Autodesk Inventor part; units mm, degrees
(part 4 of 4)
sketch "Эскиз12" plane through (0, 0, 5) normal (0, 0, 1) x (1, 0, 0)
  arc A0 (45.1929, -106.1976) -> (44.4998, -103.5049) centre (42.2719, -105.5139) ccw projected
  arc A1 (-3.3547, -38.1199) -> (-21.9349, -33.766) centre (-14.404, -43.4501) ccw projected
  line L0 (-21.9349, -33.766) -> (-22.5081, -34.2402) projected
  line L1 (-22.5081, -34.2402) -> (-23.0514, -34.7484) projected
  line L2 (-23.0514, -34.7484) -> (-23.3602, -34.9338) projected
  line L3 (-23.3602, -34.9338) -> (-23.5194, -34.9702) projected
  line L4 (-23.5194, -34.9702) -> (-23.6529, -34.9806) projected
  line L5 (-23.6529, -34.9806) -> (-23.7727, -34.9768) projected
  line L6 (-23.7727, -34.9768) -> (-23.8833, -34.9636) projected
  line L7 (-23.8833, -34.9636) -> (-24.0859, -34.9174) projected
  line L8 (-24.0859, -34.9174) -> (-24.2711, -34.8524) projected
  line L9 (-24.2711, -34.8524) -> (-24.4437, -34.7734) projected
  line L10 (-24.4437, -34.7734) -> (-24.6063, -34.683) projected
  line L11 (-24.6063, -34.683) -> (-24.9077, -34.4748) projected
  line L12 (-24.9077, -34.4748) -> (-25.1895, -34.2439) projected
  line L13 (-25.1895, -34.2439) -> (-25.5122, -34.0611) projected
  line L14 (-25.5122, -34.0611) -> (-25.8619, -33.9111) projected
  line L15 (-25.8619, -33.9111) -> (-26.2315, -33.7867) projected
  line L16 (-26.2315, -33.7867) -> (-26.6177, -33.685) projected
  line L17 (-26.6177, -33.685) -> (-27.0185, -33.6047) projected
  line L18 (-27.0185, -33.6047) -> (-27.4325, -33.5452) projected
  line L19 (-27.4325, -33.5452) -> (-27.8584, -33.5059) projected
  line L20 (-27.8584, -33.5059) -> (-28.295, -33.4867) projected
  line L21 (-28.295, -33.4867) -> (-28.7415, -33.4875) projected
  line L22 (-28.7415, -33.4875) -> (-29.0823, -33.5012) projected
  line L23 (-29.0823, -33.5012) -> (-30.1782, -35.3504) projected
  line L24 (-30.1782, -35.3504) -> (-30.0266, -35.6559) projected
  line L25 (-30.0266, -35.6559) -> (-29.813, -36.0479) projected
  line L26 (-29.813, -36.0479) -> (-29.5865, -36.4218) projected
  line L27 (-29.5865, -36.4218) -> (-29.3476, -36.7765) projected
  line L28 (-29.3476, -36.7765) -> (-29.0966, -37.111) projected
  line L29 (-29.0966, -37.111) -> (-28.8338, -37.4241) projected
  line L30 (-28.8338, -37.4241) -> (-28.5592, -37.7141) projected
  line L31 (-28.5592, -37.7141) -> (-28.2726, -37.9785) projected
  line L32 (-28.2726, -37.9785) -> (-27.9731, -38.2133) projected
  line L33 (-27.9731, -38.2133) -> (-27.6579, -38.4086) projected
  line L34 (-27.6579, -38.4086) -> (-27.32, -38.545) projected
  line L35 (-27.32, -38.545) -> (-26.9927, -38.7094) projected
  line L36 (-26.9927, -38.7094) -> (-26.8353, -38.8087) projected
  line L37 (-26.8353, -38.8087) -> (-26.6832, -38.9221) projected
  line L38 (-26.6832, -38.9221) -> (-26.5372, -39.0534) projected
  line L39 (-26.5372, -39.0534) -> (-26.3994, -39.209) projected
  line L40 (-26.3994, -39.209) -> (-26.3347, -39.2997) projected
  line L41 (-26.3347, -39.2997) -> (-26.2739, -39.4029) projected
  line L42 (-26.2739, -39.4029) -> (-26.2189, -39.5249) projected
  line L43 (-26.2189, -39.5249) -> (-26.1744, -39.6821) projected
  line L44 (-26.1744, -39.6821) -> (-26.1888, -40.0421) projected
  line L45 (-26.1888, -40.0421) -> (-26.3737, -40.7626) projected
  line L46 (-26.3737, -40.7626) -> (-26.5146, -41.493) projected
  line L47 (-26.5146, -41.493) -> (-26.6554, -41.8246) projected
  line L48 (-26.6554, -41.8246) -> (-26.7629, -41.9477) projected
  line L49 (-26.7629, -41.9477) -> (-26.8648, -42.0345) projected
  line L50 (-26.8648, -42.0345) -> (-26.9639, -42.1018) projected
  line L51 (-26.9639, -42.1018) -> (-27.0611, -42.1561) projected
  line L52 (-27.0611, -42.1561) -> (-27.2522, -42.2379) projected
  line L53 (-27.2522, -42.2379) -> (-27.4403, -42.2942) projected
  line L54 (-27.4403, -42.2942) -> (-27.6263, -42.3317) projected
  line L55 (-27.6263, -42.3317) -> (-27.811, -42.3542) projected
  line L56 (-27.811, -42.3542) -> (-28.1772, -42.3629) projected
  line L57 (-28.1772, -42.3629) -> (-28.5409, -42.3417) projected
  line L58 (-28.5409, -42.3417) -> (-28.9094, -42.3835) projected
  line L59 (-28.9094, -42.3835) -> (-29.2805, -42.4677) projected
  line L60 (-29.2805, -42.4677) -> (-29.6526, -42.5842) projected
  line L61 (-29.6526, -42.5842) -> (-30.0249, -42.729) projected
  line L62 (-30.0249, -42.729) -> (-30.3963, -42.8997) projected
  line L63 (-30.3963, -42.8997) -> (-30.7662, -43.0948) projected
  line L64 (-30.7662, -43.0948) -> (-31.1338, -43.3134) projected
  line L65 (-31.1338, -43.3134) -> (-31.4984, -43.5545) projected
  line L66 (-31.4984, -43.5545) -> (-31.8591, -43.8176) projected
  line L67 (-31.8591, -43.8176) -> (-32.1268, -44.029) projected
  line L68 (-32.1268, -44.029) -> (-31.9265, -46.1692) projected
  line L69 (-31.9265, -46.1692) -> (-31.6243, -46.3272) projected
  line L70 (-31.6243, -46.3272) -> (-31.221, -46.5188) projected
  line L71 (-31.221, -46.5188) -> (-30.8181, -46.6881) projected
  line L72 (-30.8181, -46.6881) -> (-30.4163, -46.8347) projected
  line L73 (-30.4163, -46.8347) -> (-30.0166, -46.9578) projected
  line L74 (-30.0166, -46.9578) -> (-29.6199, -47.0566) projected
  line L75 (-29.6199, -47.0566) -> (-29.2273, -47.1298) projected
  line L76 (-29.2273, -47.1298) -> (-28.84, -47.1753) projected
  line L77 (-28.84, -47.1753) -> (-28.4598, -47.1892) projected
  line L78 (-28.4598, -47.1892) -> (-28.0899, -47.1619) projected
  line L79 (-28.0899, -47.1619) -> (-27.7364, -47.0736) projected
  line L80 (-27.7364, -47.0736) -> (-27.3749, -47.0142) projected
  line L81 (-27.3749, -47.0142) -> (-27.1893, -47.0021) projected
  line L82 (-27.1893, -47.0021) -> (-26.9995, -47.0044) projected
  line L83 (-26.9995, -47.0044) -> (-26.8043, -47.0248) projected
  line L84 (-26.8043, -47.0248) -> (-26.6014, -47.0697) projected
  line L85 (-26.6014, -47.0697) -> (-26.4957, -47.1051) projected
  line L86 (-26.4957, -47.1051) -> (-26.3859, -47.1528) projected
  line L87 (-26.3859, -47.1528) -> (-26.2696, -47.2192) projected
  line L88 (-26.2696, -47.2192) -> (-26.1412, -47.3202) projected
  line L89 (-26.1412, -47.3202) -> (-25.9413, -47.6199) projected
  line L90 (-25.9413, -47.6199) -> (-25.6674, -48.3115) projected
  line L91 (-25.6674, -48.3115) -> (-25.352, -48.9853) projected
  line L92 (-25.352, -48.9853) -> (-25.2711, -49.3363) projected
  line L93 (-25.2711, -49.3363) -> (-25.2857, -49.499) projected
  line L94 (-25.2857, -49.499) -> (-25.3171, -49.6291) projected
  line L95 (-25.3171, -49.6291) -> (-25.3576, -49.7418) projected
  line L96 (-25.3576, -49.7418) -> (-25.4044, -49.8429) projected
  line L97 (-25.4044, -49.8429) -> (-25.5109, -50.0214) projected
  line L98 (-25.5109, -50.0214) -> (-25.63, -50.1775) projected
  line L99 (-25.63, -50.1775) -> (-25.7585, -50.3172) projected
  line L100 (-25.7585, -50.3172) -> (-25.8946, -50.4439) projected
  line L101 (-25.8946, -50.4439) -> (-26.1858, -50.6662) projected
  line L102 (-26.1858, -50.6662) -> (-26.4925, -50.8629) projected
  line L103 (-26.4925, -50.8629) -> (-26.7661, -51.1133) projected
  line L104 (-26.7661, -51.1133) -> (-27.0168, -51.3996) projected
  line L105 (-27.0168, -51.3996) -> (-27.2493, -51.7125) projected
  line L106 (-27.2493, -51.7125) -> (-27.4654, -52.0484) projected
  line L107 (-27.4654, -52.0484) -> (-27.6656, -52.4049) projected
  line L108 (-27.6656, -52.4049) -> (-27.8501, -52.7802) projected
  line L109 (-27.8501, -52.7802) -> (-28.0191, -53.1731) projected
  line L110 (-28.0191, -53.1731) -> (-28.1723, -53.5824) projected
  line L111 (-28.1723, -53.5824) -> (-28.3095, -54.0073) projected
  line L112 (-28.3095, -54.0073) -> (-28.4018, -54.3356) projected
  line L113 (-28.4018, -54.3356) -> (-26.9818, -55.9493) projected
  line L114 (-26.9818, -55.9493) -> (-26.6444, -55.8996) projected
  line L115 (-26.6444, -55.8996) -> (-26.2055, -55.8175) projected
  line L116 (-26.2055, -55.8175) -> (-25.78, -55.7177) projected
  line L117 (-25.78, -55.7177) -> (-25.3688, -55.6001) projected
  line L118 (-25.3688, -55.6001) -> (-24.9731, -55.4648) projected
  line L119 (-24.9731, -55.4648) -> (-24.5941, -55.3116) projected
  line L120 (-24.5941, -55.3116) -> (-24.2334, -55.14) projected
  line L121 (-24.2334, -55.14) -> (-23.8934, -54.9491) projected
  line L122 (-23.8934, -54.9491) -> (-23.5776, -54.7369) projected
  line L123 (-23.5776, -54.7369) -> (-23.2944, -54.4974) projected
  line L124 (-23.2944, -54.4974) -> (-23.0603, -54.2182) projected
  line L125 (-23.0603, -54.2182) -> (-22.8028, -53.9577) projected
  line L126 (-22.8028, -53.9577) -> (-22.6598, -53.8387) projected
  line L127 (-22.6598, -53.8387) -> (-22.5048, -53.7291) projected
  line L128 (-22.5048, -53.7291) -> (-22.3349, -53.6308) projected
  line L129 (-22.3349, -53.6308) -> (-22.1443, -53.5479) projected
  line L130 (-22.1443, -53.5479) -> (-22.0381, -53.5144) projected
  line L131 (-22.0381, -53.5144) -> (-21.9211, -53.4885) projected
  line L132 (-21.9211, -53.4885) -> (-21.788, -53.4739) projected
  line L133 (-21.788, -53.4739) -> (-21.6248, -53.4801) projected
  line L134 (-21.6248, -53.4801) -> (-21.2869, -53.605) projected
  line L135 (-21.2869, -53.605) -> (-20.6588, -54.0036) projected
  line L136 (-20.6588, -54.0036) -> (-20.0076, -54.3632) projected
  line L137 (-20.0076, -54.3632) -> (-19.7358, -54.5996) projected
  line L138 (-19.7358, -54.5996) -> (-19.652, -54.7398) projected
  line L139 (-19.652, -54.7398) -> (-19.6009, -54.8636) projected
  line L140 (-19.6009, -54.8636) -> (-19.5675, -54.9786) projected
  line L141 (-19.5675, -54.9786) -> (-19.5459, -55.0879) projected
  line L142 (-19.5459, -55.0879) -> (-19.5272, -55.2949) projected
  line L143 (-19.5272, -55.2949) -> (-19.5318, -55.4911) projected
  line L144 (-19.5318, -55.4911) -> (-19.5536, -55.6797) projected
  line L145 (-19.5536, -55.6797) -> (-19.5893, -55.8623) projected
  line L146 (-19.5893, -55.8623) -> (-19.6941, -56.2132) projected
  line L147 (-19.6941, -56.2132) -> (-19.8267, -56.5526) projected
  line L148 (-19.8267, -56.5526) -> (-19.9008, -56.916) projected
  line L149 (-19.9008, -56.916) -> (-19.9354, -57.2949) projected
  line L150 (-19.9354, -57.2949) -> (-19.9396, -57.6849) projected
  line L151 (-19.9396, -57.6849) -> (-19.9169, -58.0836) projected
  line L152 (-19.9169, -58.0836) -> (-19.8694, -58.4897) projected
  line L153 (-19.8694, -58.4897) -> (-19.7981, -58.9018) projected
  line L154 (-19.7981, -58.9018) -> (-19.7038, -59.3189) projected
  line L155 (-19.7038, -59.3189) -> (-19.5871, -59.7401) projected
  line L156 (-19.5871, -59.7401) -> (-19.4484, -60.1645) projected
  line L157 (-19.4484, -60.1645) -> (-19.3301, -60.4844) projected
  line L158 (-19.3301, -60.4844) -> (-17.2328, -60.9553) projected
  line L159 (-17.2328, -60.9553) -> (-16.989, -60.7167) projected
  line L160 (-16.989, -60.7167) -> (-16.6822, -60.3923) projected
  line L161 (-16.6822, -60.3923) -> (-16.3967, -60.0614) projected
  line L162 (-16.3967, -60.0614) -> (-16.1331, -59.7246) projected
  line L163 (-16.1331, -59.7246) -> (-15.8925, -59.3825) projected
  line L164 (-15.8925, -59.3825) -> (-15.676, -59.0358) projected
  line L165 (-15.676, -59.0358) -> (-15.485, -58.685) projected
  line L166 (-15.485, -58.685) -> (-15.3221, -58.3307) projected
  line L167 (-15.3221, -58.3307) -> (-15.1914, -57.9734) projected
  line L168 (-15.1914, -57.9734) -> (-15.103, -57.6132) projected
  line L169 (-15.103, -57.6132) -> (-15.0777, -57.2497) projected
  line L170 (-15.0777, -57.2497) -> (-15.0225, -56.8876) projected
  line L171 (-15.0225, -56.8876) -> (-14.9767, -56.7073) projected
  line L172 (-14.9767, -56.7073) -> (-14.9159, -56.5275) projected
  line L173 (-14.9159, -56.5275) -> (-14.8361, -56.3481) projected
  line L174 (-14.8361, -56.3481) -> (-14.7307, -56.169) projected
  line L175 (-14.7307, -56.169) -> (-14.6645, -56.0795) projected
  line L176 (-14.6645, -56.0795) -> (-14.5851, -55.9898) projected
  line L177 (-14.5851, -55.9898) -> (-14.486, -55.8997) projected
  line L178 (-14.486, -55.8997) -> (-14.3503, -55.8088) projected
  line L179 (-14.3503, -55.8088) -> (-14.0035, -55.7113) projected
  line L180 (-14.0035, -55.7113) -> (-13.2611, -55.6645) projected
  arc A2 (41.85, -107.2531) -> (41.1568, -104.5603) centre (38.9289, -106.5694) ccw projected
  line L181 (41.85, -107.2531) -> (36.907, -128.3716) projected
  line L182 (36.907, -128.3716) -> (40.0869, -128.0131) projected
  line L183 (40.0869, -128.0131) -> (45.1929, -106.1976) projected
  circle A3 centre (-14.404, -43.4501) radius 2.5 projected
  circle A4 centre (-8.4487, -38.1084) radius 1.6 projected
  circle A5 centre (-19.7457, -37.4948) radius 1.6 projected
  circle A6 centre (-20.3593, -48.7918) radius 1.6 projected
  circle A7 centre (-9.0623, -49.4054) radius 1.6 projected
  circle A8 centre (-39.9568, -59.168) radius 2.5 projected
  line L184 (-39.9568, -59.168) -> (-14.404, -43.4501)
  line L185 (-27.1804, -51.309) -> (27.0799, -139.521)
  arc A9 (-12.9217, -138.8256) -> (-10.8309, -140.6586) centre (-10.1237, -137.7432) ccw
  line L186 (-12.9217, -138.8256) -> (-34.4952, -83.0601)
  arc A10 (-34.4952, -83.0601) -> (-45.9439, -69.8756) centre (-58.5108, -92.3508) ccw
  arc A11 (-29.9854, -66.3142) -> (-30.1782, -85.3794) centre (-6.1627, -76.0887) ccw
  line L187 (-30.1782, -85.3794) -> (-10.472, -136.3179)
  arc A12 (-10.472, -136.3179) -> (-8.3812, -138.1509) centre (-7.6741, -135.2355) ccw
  line L188 (-8.3812, -138.1509) -> (12.6969, -143.2636)
  line L189 (12.6969, -143.2636) -> (10.9428, -145.94)
  line L190 (10.9428, -145.94) -> (-10.8309, -140.6586)
  circle A13 centre (-47.4326, -62.0164) radius 1.6 projected
  circle A14 centre (-37.1084, -66.6437) radius 1.6 projected
  circle A15 centre (-32.4811, -56.3196) radius 1.6 projected
  circle A16 centre (-39.9568, -59.168) radius 2.5 projected
  circle A17 centre (-42.8052, -51.6922) radius 1.6 projected
  arc A18 (-41.4259, -46.9885) -> (-28.2942, -62.9735) centre (-39.9568, -59.168) ccw projected
  line L191 (-28.085, -62.2597) -> (-28.2942, -62.9735) projected
  line L192 (-27.9195, -61.5344) -> (-28.085, -62.2597) projected
  line L193 (-27.7675, -61.2078) -> (-27.9195, -61.5344) projected
  line L194 (-27.6559, -61.0885) -> (-27.7675, -61.2078) projected
  line L195 (-27.5511, -61.0052) -> (-27.6559, -61.0885) projected
  line L196 (-27.4498, -60.9413) -> (-27.5511, -61.0052) projected
  line L197 (-27.3508, -60.8903) -> (-27.4498, -60.9413) projected
  line L198 (-27.1571, -60.815) -> (-27.3508, -60.8903) projected
  line L199 (-26.9672, -60.7651) -> (-27.1571, -60.815) projected
  line L200 (-26.78, -60.734) -> (-26.9672, -60.7651) projected
  line L201 (-26.5947, -60.7178) -> (-26.78, -60.734) projected
  line L202 (-26.2284, -60.7215) -> (-26.5947, -60.7178) projected
  line L203 (-25.8656, -60.755) -> (-26.2284, -60.7215) projected
  line L204 (-25.4958, -60.7256) -> (-25.8656, -60.755) projected
  line L205 (-25.1221, -60.6541) -> (-25.4958, -60.7256) projected
  line L206 (-24.7463, -60.5502) -> (-25.1221, -60.6541) projected
  line L207 (-24.3693, -60.4182) -> (-24.7463, -60.5502) projected
  line L208 (-23.9923, -60.2602) -> (-24.3693, -60.4182) projected
  line L209 (-23.616, -60.0777) -> (-23.9923, -60.2602) projected
  line L210 (-23.2412, -59.8717) -> (-23.616, -60.0777) projected
  line L211 (-22.8687, -59.6431) -> (-23.2412, -59.8717) projected
  line L212 (-22.4992, -59.3924) -> (-22.8687, -59.6431) projected
  line L213 (-22.2246, -59.1902) -> (-22.4992, -59.3924) projected
  line L214 (-22.3522, -57.0445) -> (-22.2246, -59.1902) projected
  line L215 (-22.6489, -56.8763) -> (-22.3522, -57.0445) projected
  line L216 (-23.0454, -56.6711) -> (-22.6489, -56.8763) projected
  line L217 (-23.4424, -56.4882) -> (-23.0454, -56.6711) projected
  line L218 (-23.839, -56.3281) -> (-23.4424, -56.4882) projected
  line L219 (-24.2343, -56.1915) -> (-23.839, -56.3281) projected
  line L220 (-24.6274, -56.0793) -> (-24.2343, -56.1915) projected
  line L221 (-25.0173, -55.9929) -> (-24.6274, -56.0793) projected
  line L222 (-25.4028, -55.9343) -> (-25.0173, -55.9929) projected
  line L223 (-25.7823, -55.9075) -> (-25.4028, -55.9343) projected
  line L224 (-26.153, -55.9222) -> (-25.7823, -55.9075) projected
  line L225 (-26.5093, -55.9985) -> (-26.153, -55.9222) projected
  line L226 (-26.8725, -56.0456) -> (-26.5093, -55.9985) projected
  line L227 (-27.0584, -56.0515) -> (-26.8725, -56.0456) projected
  line L228 (-27.248, -56.0427) -> (-27.0584, -56.0515) projected
  line L229 (-27.4425, -56.0157) -> (-27.248, -56.0427) projected
  line L230 (-27.6437, -55.9639) -> (-27.4425, -56.0157) projected
  line L231 (-27.7481, -55.925) -> (-27.6437, -55.9639) projected
  line L232 (-27.8563, -55.8736) -> (-27.7481, -55.925) projected
  line L233 (-27.9702, -55.8032) -> (-27.8563, -55.8736) projected
  line L234 (-28.0951, -55.698) -> (-27.9702, -55.8032) projected
  line L235 (-28.2847, -55.3917) -> (-28.0951, -55.698) projected
  line L236 (-28.5351, -54.6912) -> (-28.2847, -55.3917) projected
  line L237 (-28.8274, -54.0071) -> (-28.5351, -54.6912) projected
  line L238 (-28.8965, -53.6536) -> (-28.8274, -54.0071) projected
  line L239 (-28.8763, -53.4914) -> (-28.8965, -53.6536) projected
  line L240 (-28.8405, -53.3624) -> (-28.8763, -53.4914) projected
  line L241 (-28.7962, -53.2512) -> (-28.8405, -53.3624) projected
  line L242 (-28.746, -53.1517) -> (-28.7962, -53.2512) projected
  line L243 (-28.6335, -52.977) -> (-28.746, -53.1517) projected
  line L244 (-28.5092, -52.825) -> (-28.6335, -52.977) projected
  line L245 (-28.3761, -52.6897) -> (-28.5092, -52.825) projected
  line L246 (-28.2357, -52.5677) -> (-28.3761, -52.6897) projected
  line L247 (-27.9372, -52.3554) -> (-28.2357, -52.5677) projected
  line L248 (-27.624, -52.1693) -> (-27.9372, -52.3554) projected
  line L249 (-27.3421, -51.9282) -> (-27.624, -52.1693) projected
  line L250 (-27.0818, -51.6507) -> (-27.3421, -51.9282) projected
  line L251 (-26.8388, -51.3457) -> (-27.0818, -51.6507) projected
  line L252 (-26.6114, -51.0173) -> (-26.8388, -51.3457) projected
  line L253 (-26.3993, -50.6679) -> (-26.6114, -51.0173) projected
  line L254 (-26.2021, -50.2991) -> (-26.3993, -50.6679) projected
  line L255 (-26.02, -49.9121) -> (-26.2021, -50.2991) projected
  line L256 (-25.853, -49.5082) -> (-26.02, -49.9121) projected
  line L257 (-25.7014, -49.0882) -> (-25.853, -49.5082) projected
  line L258 (-25.5981, -48.7632) -> (-25.7014, -49.0882) projected
  line L259 (-25.5981, -48.7632) -> (-26.9625, -47.1023) projected
  line L260 (-27.3014, -47.1406) -> (-26.9625, -47.1023) projected
  line L261 (-27.7429, -47.2077) -> (-27.3014, -47.1406) projected
  line L262 (-28.1715, -47.2931) -> (-27.7429, -47.2077) projected
  line L263 (-28.5864, -47.3967) -> (-28.1715, -47.2931) projected
  line L264 (-28.9865, -47.5185) -> (-28.5864, -47.3967) projected
  line L265 (-29.3705, -47.6588) -> (-28.9865, -47.5185) projected
  line L266 (-29.7368, -47.818) -> (-29.3705, -47.6588) projected
  line L267 (-30.0831, -47.9973) -> (-29.7368, -47.818) projected
  line L268 (-30.4059, -48.1987) -> (-30.0831, -47.9973) projected
  line L269 (-30.6971, -48.4284) -> (-30.4059, -48.1987) projected
  line L270 (-30.9405, -48.6995) -> (-30.6971, -48.4284) projected
  line L271 (-31.2067, -48.9511) -> (-30.9405, -48.6995) projected
  line L272 (-31.3536, -49.0652) -> (-31.2067, -48.9511) projected
  line L273 (-31.5122, -49.1695) -> (-31.3536, -49.0652) projected
  line L274 (-31.6854, -49.262) -> (-31.5122, -49.1695) projected
  line L275 (-31.8786, -49.3384) -> (-31.6854, -49.262) projected
  line L276 (-31.986, -49.3683) -> (-31.8786, -49.3384) projected
  line L277 (-32.1037, -49.3902) -> (-31.986, -49.3683) projected
  line L278 (-32.2372, -49.4003) -> (-32.1037, -49.3902) projected
  line L279 (-32.4002, -49.3886) -> (-32.2372, -49.4003) projected
  line L280 (-32.7336, -49.2522) -> (-32.4002, -49.3886) projected
  line L281 (-33.3479, -48.8326) -> (-32.7336, -49.2522) projected
  line L282 (-33.9864, -48.4511) -> (-33.3479, -48.8326) projected
  line L283 (-34.2501, -48.2056) -> (-33.9864, -48.4511) projected
  line L284 (-34.3291, -48.0626) -> (-34.2501, -48.2056) projected
  line L285 (-34.376, -47.9372) -> (-34.3291, -48.0626) projected
  line L286 (-34.4055, -47.8211) -> (-34.376, -47.9372) projected
  line L287 (-34.4234, -47.7112) -> (-34.4055, -47.8211) projected
  line L288 (-34.4351, -47.5037) -> (-34.4234, -47.7112) projected
  line L289 (-34.4238, -47.3077) -> (-34.4351, -47.5037) projected
  line L290 (-34.3956, -47.12) -> (-34.4238, -47.3077) projected
  line L291 (-34.3538, -46.9387) -> (-34.3956, -47.12) projected
  line L292 (-34.237, -46.5916) -> (-34.3538, -46.9387) projected
  line L293 (-34.0931, -46.2568) -> (-34.237, -46.5916) projected
  line L294 (-34.0067, -45.8961) -> (-34.0931, -46.2568) projected
  line L295 (-33.9593, -45.5186) -> (-34.0067, -45.8961) projected
  line L296 (-33.9419, -45.129) -> (-33.9593, -45.5186) projected
  line L297 (-33.951, -44.7298) -> (-33.9419, -45.129) projected
  line L298 (-33.9848, -44.3224) -> (-33.951, -44.7298) projected
  line L299 (-34.0421, -43.9081) -> (-33.9848, -44.3224) projected
  line L300 (-34.1221, -43.488) -> (-34.0421, -43.9081) projected
  line L301 (-34.2244, -43.063) -> (-34.1221, -43.488) projected
  line L302 (-34.3487, -42.6342) -> (-34.2244, -43.063) projected
  line L303 (-34.4561, -42.3105) -> (-34.3487, -42.6342) projected
  line L304 (-36.5363, -41.7688) -> (-34.4561, -42.3105) projected
  line L305 (-36.7879, -41.999) -> (-36.5363, -41.7688) projected
  line L306 (-37.1056, -42.3127) -> (-36.7879, -41.999) projected
  line L307 (-37.4022, -42.6338) -> (-37.1056, -42.3127) projected
  line L308 (-37.677, -42.9614) -> (-37.4022, -42.6338) projected
  line L309 (-37.9291, -43.2952) -> (-37.677, -42.9614) projected
  line L310 (-38.1573, -43.6344) -> (-37.9291, -43.2952) projected
  line L311 (-38.36, -43.9785) -> (-38.1573, -43.6344) projected
  line L312 (-38.5348, -44.327) -> (-38.36, -43.9785) projected
  line L313 (-38.6775, -44.6797) -> (-38.5348, -44.327) projected
  line L314 (-38.7781, -45.0367) -> (-38.6775, -44.6797) projected
  line L315 (-38.8157, -45.3992) -> (-38.7781, -45.0367) projected
  line L316 (-38.8831, -45.7592) -> (-38.8157, -45.3992) projected
  line L317 (-38.935, -45.9378) -> (-38.8831, -45.7592) projected
  line L318 (-39.0019, -46.1155) -> (-38.935, -45.9378) projected
  line L319 (-39.0877, -46.292) -> (-39.0019, -46.1155) projected
  line L320 (-39.1991, -46.4674) -> (-39.0877, -46.292) projected
  line L321 (-39.2684, -46.5547) -> (-39.1991, -46.4674) projected
  line L322 (-39.3507, -46.6417) -> (-39.2684, -46.5547) projected
  line L323 (-39.4528, -46.7283) -> (-39.3507, -46.6417) projected
  line L324 (-39.5916, -46.8146) -> (-39.4528, -46.7283) projected
  line L325 (-39.9414, -46.9002) -> (-39.5916, -46.8146) projected
  line L326 (-40.685, -46.9219) -> (-39.9414, -46.9002) projected
  line L327 (-41.4259, -46.9885) -> (-40.685, -46.9219) projected
  line L328 (44.4998, -103.5049) -> (6.7267, -54.4578) projected
  arc A19 (-3.3547, -38.1199) -> (6.7267, -54.4578) centre (80.4084, 2.2873) ccw projected
  arc A20 (-10.9612, -56.9979) -> (-13.2611, -55.6645) centre (-15.1743, -61.6145) ccw projected
  line L329 (-10.9612, -56.9979) -> (41.1568, -104.5603) projected
  point P0 (0, 0)
  point P1 (-29.9854, -66.3142)
  point P2 (-45.9391, -69.8783)
  constraints: 14 end point, 8 point on circle, 6 symmetric about line, 4 centre point, 1 midpoint, 1 perpendicular, 2 other
extrude "Выдавливание12" add sketch "Эскиз12" against normal up to surface (5 mm away) contours A11 L187 A12 L188 L189 L190 A9 L186 A10 A18
